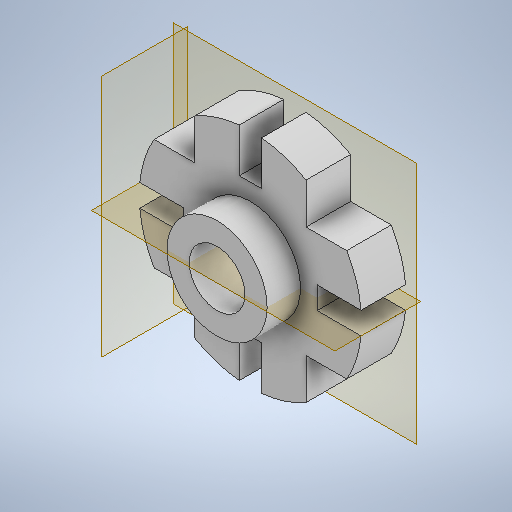
# Autodesk Inventor part: ch3ex5
Saved by Autodesk Inventor 2025.2 (Build 292293000, 293)
## iProperties
Created: 2025-02-01
Part Number: ch3ex5
Material: Generic
Document SubType Name: Modeling
Designer: Moofin
Density: 1 g/cm^3
Appearance: Default
Author: Moofin
Autodesk Inventor part; units mm, degrees
sketch "Sketch1" plane through (0, 0, 0) normal (0, 0, 1) x (1, 0, 0)
  circle A0 centre (63.5, 0) radius 63.5
  line L0 (-25.4, 0) -> (152.4, 0) projected
  line L1 (0, 88.9) -> (0, -88.9) projected
  point P0 (0, 0)
  dimension "d0" = 127
  dimension "d1" = 0
  dimension "d2" = 63.5
  constraints: 1 centre point
  measures "d0" diameter of A0
  measures "d1" distance from line of L0 A0.centre
  measures "d2" distance from line of L1 A0.centre
extrude "Extrusion1" add sketch "Sketch1" along normal blind 25.4
sketch "Sketch2" plane through (0, 0, 0) normal (0, 0, 1) x (1, 0, 0)
  circle A0 centre (63.5, 0) radius 28.575
  line L0 (0, 40.005) -> (0, -40.005) projected
  line L1 (-18.415, 0) -> (110.49, 0) projected
  point P0 (0, 0)
  dimension "d5" = 57.15
  dimension "d6" = 63.5
  dimension "d7" = 0
  constraints: 1 centre point
  measures "d5" diameter of A0
  measures "d6" distance from line of L0 A0.centre
  measures "d7" distance from line of L1 A0.centre
extrude "Extrusion2" add sketch "Sketch2" along normal blind 44.45
sketch "Sketch3" plane through (63.5, 0, 44.45) normal (0, 0, 1) x (1, 0, 0)
  circle A0 centre (0, 0) radius 28.575 projected
  point P0 (-63.5, 0)
  constraints: 1 coincident
hole "Hole1" at (63.5, 0, 44.45) direction (0, 0, -1) diameter 31.75 end through all
sketch "Sketch4" plane through (63.5, 0, 25.4) normal (0, 0, 1) x (1, 0, 0)
  line L0 (-6.35, 63.5) -> (6.35, 63.5)
  line L1 (6.35, 63.5) -> (6.35, 38.1)
  line L2 (6.35, 38.1) -> (-6.35, 38.1)
  line L3 (-6.35, 38.1) -> (-6.35, 63.5)
  circle A0 centre (0, 0) radius 63.5 projected
  line L4 (-63.5, 6.35) -> (-38.1, 6.35)
  line L5 (-38.1, 6.35) -> (-38.1, -6.35)
  line L6 (-38.1, -6.35) -> (-63.5, -6.35)
  line L7 (-63.5, -6.35) -> (-63.5, 6.35)
  line L8 (-6.35, -38.1) -> (6.35, -38.1)
  line L9 (6.35, -38.1) -> (6.35, -63.5)
  line L10 (6.35, -63.5) -> (-6.35, -63.5)
  line L11 (-6.35, -63.5) -> (-6.35, -38.1)
  line L12 (38.1, 6.35) -> (63.5, 6.35)
  line L13 (63.5, 6.35) -> (63.5, -6.35)
  line L14 (63.5, -6.35) -> (38.1, -6.35)
  line L15 (38.1, -6.35) -> (38.1, 6.35)
  point P0 (-63.5, 0)
  point P1 (6.35, 50.8)
  point P2 (0, 38.1)
  point P3 (-63.1817, 6.35)
  point P4 (-63.1817, -6.35)
  point P5 (-6.35, -63.1817)
  point P6 (6.35, -63.1817)
  point P7 (63.1817, -6.35)
  point P8 (63.1817, 6.35)
  point P9 (6.35, 63.1817)
  point P10 (-6.35, 63.1817)
  dimension "d17" = 12.7
  dimension "d18" = 25.4
  dimension "d19" = 38.1
  dimension "d20" = 6.35
  dimension "d21" = 25.4
  dimension "d22" = 12.7
  dimension "d23" = 38.1
  dimension "d24" = 6.35
  dimension "d25" = 25.4
  dimension "d26" = 12.7
  dimension "d27" = 6.35
  dimension "d28" = 38.1
  dimension "d29" = 25.4
  dimension "d30" = 12.7
  dimension "d31" = 6.35
  dimension "d32" = 38.1
  constraints: 32 end point, 8 parallel, 4 horizontal, 4 perpendicular, 2 midpoint, 1 other
  measures "d17" distance from line of point (6.35, 50.8) L3
  measures "d18" distance from line of point (0, 38.1) L0
  measures "d19" distance from line of point (0, 0) L2
  measures "d20" distance from line of point (0, 0) L3
  measures "d21" distance between parallel lines of L5 L7
  measures "d22" distance between parallel lines of L6 L4
  measures "d23" distance from line of point (0, 0) L5
  measures "d24" distance from line of point (0, 0) L6
  measures "d25" distance between parallel lines of L10 L8
  measures "d26" distance between parallel lines of L9 L11
  measures "d27" distance from line of point (0, 0) L11
  measures "d28" distance from line of point (0, 0) L8
  measures "d29" distance between parallel lines of L13 L15
  measures "d30" distance between parallel lines of L14 L12
  measures "d31" distance from line of point (0, 0) L14
  measures "d32" distance from line of point (0, 0) L15
extrude "Extrusion3" cut sketch "Sketch4" against normal up to surface (25.4 mm away) contours A0 L1 L2 L3 | L4 L5 L6 A0 | A0 L14 L15 L12 | L11 L8 L9 A0
sketch "Sketch5" plane through (0, 0, 25.4) normal (0, 0, 1) x (1, 0, 0)
  line L0 (95.25, 64.7866) -> (128.2866, 64.7866)
  line L1 (128.2866, 64.7866) -> (128.2866, 31.75)
  line L2 (128.2866, 31.75) -> (95.25, 31.75)
  line L3 (95.25, 31.75) -> (95.25, 64.7866)
  line L4 (-25.758, 0) -> (154.5482, 0) projected
  line L5 (69.85, 63.1817) -> (69.85, 38.1) projected
  line L6 (-1.2866, 64.7866) -> (31.75, 64.7866)
  line L7 (31.75, 64.7866) -> (31.75, 31.75)
  line L8 (31.75, 31.75) -> (-1.2866, 31.75)
  line L9 (-1.2866, 31.75) -> (-1.2866, 64.7866)
  line L10 (57.15, 38.1) -> (57.15, 63.1817) projected
  line L11 (95.25, -31.75) -> (128.2866, -31.75)
  line L12 (128.2866, -31.75) -> (128.2866, -64.7866)
  line L13 (128.2866, -64.7866) -> (95.25, -64.7866)
  line L14 (95.25, -64.7866) -> (95.25, -31.75)
  line L15 (69.85, -38.1) -> (69.85, -63.1817) projected
  line L16 (31.75, -31.75) -> (-1.2866, -31.75)
  line L17 (-1.2866, -31.75) -> (-1.2866, -64.7866)
  line L18 (-1.2866, -64.7866) -> (31.75, -64.7866)
  line L19 (31.75, -64.7866) -> (31.75, -31.75)
  line L20 (57.15, -63.1817) -> (57.15, -38.1) projected
  point P0 (0, 0)
  dimension "d35" = 31.75
  dimension "d36" = 25.4
  dimension "d37" = 25.4
  dimension "d38" = 31.75
  dimension "d39" = 25.4
  dimension "d40" = 31.75
  dimension "d41" = 31.75
  dimension "d42" = 25.4
  constraints: 32 end point, 8 parallel, 7 equal length, 4 horizontal, 4 perpendicular
  measures "d35" distance between parallel lines of L4 L2
  measures "d36" distance between parallel lines of L5 L3
  measures "d37" distance between parallel lines of L10 L7
  measures "d38" distance between parallel lines of L4 L8
  measures "d39" distance between parallel lines of L15 L14
  measures "d40" distance between parallel lines of L4 L11
  measures "d41" distance between parallel lines of L4 L16
  measures "d42" distance between parallel lines of L19 L20
extrude "Extrusion4" cut sketch "Sketch5" against normal up to surface (25.4 mm away)
equation "\"d20\" = 0.5 * d17"
equation "\"d21\" = d18"
equation "\"d22\" = d17"
equation "\"d23\" = d19"
equation "\"d24\" = 0.5 * d17"
equation "\"d25\" = d18"
equation "\"d26\" = d17"
equation "\"d27\" = 0.5 * d17"
equation "\"d28\" = d19"
equation "\"d29\" = d18"
equation "\"d30\" = d17"
equation "\"d31\" = 0.5 * d17"
equation "\"d32\" = d19"
equation "\"d37\" = d36"
equation "\"d38\" = d35"
equation "\"d39\" = d36"
equation "\"d40\" = d35"
equation "\"d41\" = d35"
equation "\"d42\" = d36"
body "Solid1"
